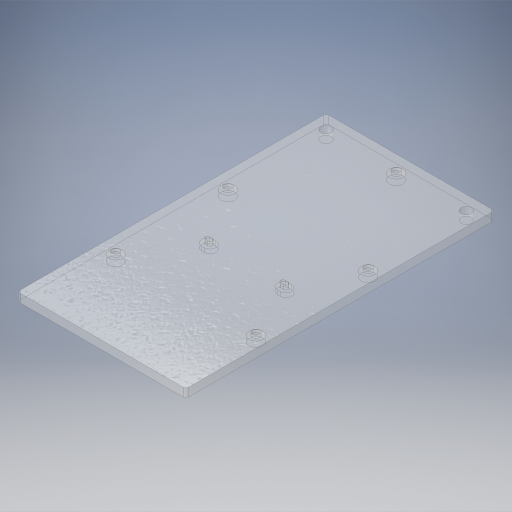
# Autodesk Inventor part: BT005_trajan20_21
Saved by Autodesk Inventor 2023 (Build 270158000, 158)
## iProperties
Company: HTBLA Kaindorf
RuleStatus: InUse
Created: 2022-08-07
Part Number: BT005_trajan20_21
Project: Zeichenmaschine_v2
Material: Acryl
Description: getriebemotor platte unten
Document SubType Name: Modeling
Designer: trajan20
Density: 1.188 g/cm^3
Appearance: Transparent - farblos
Mass: 184.772 g
Surface Area: 577.283 cm^2
Volume: 155.532 cm^3
AfterDocNew0: iProperties-Editor_aufrufen
Author: jan
Keywords: 2021
Autodesk Inventor part; units mm, degrees
ref_plane "YZ Plane" through (0, 0, 0) normal (1, 0, 0) x (0, 1, 0)
sketch "Skizze3" plane through (0, 0, 0) normal (0, 0, 1) x (1, 0, 0)
  line L0 (0, 0) -> (-220, 0)
  line L1 (-220, 0) -> (-220, 120)
  line L2 (-220, 120) -> (0, 120)
  line L3 (0, 120) -> (0, 0)
  point P0 (-210, 60)
  point P1 (-140, 10)
  point P2 (-140, 110)
  point P3 (-220, 60)
  point P4 (-60, 10)
  point P5 (-60, 110)
  point P6 (-210, 10)
  point P7 (-210, 110)
  dimension "d4" = 120
  dimension "d5" = 220
  dimension "d31" = 10
  dimension "d32" = 10
  dimension "d33" = 10
  dimension "d34" = 80
  dimension "d42" = 60
  constraints: 8 end point, 5 horizontal alignment, 4 vertical alignment, 2 parallel, 1 horizontal, 1 midpoint, 1 perpendicular
  measures "d4" distance between parallel lines of L0 L2
  measures "d5" distance between parallel lines of L1 L3
  measures "d31" distance from line of L1 point (-210, 60)
  measures "d32" distance from line of point (-140, 110) L2
  measures "d33" distance from line of L0 point (-140, 10)
  measures "d34" distance from line of L1 point (-140, 10)
  measures "d42" distance from line of L3 point (-60, 110)
extrude "Extrusion3" add sketch "Skizze3" along normal blind 6
ref_plane "Arbeitsebene1" through (-110, 120, 6) normal (-1, 0, 0) x (0, -1, 0)
ref_plane "Arbeitsebene2" through (-220, 60, 6) normal (0, -1, 0) x (1, 0, 0)
fillet "Rundung2" radius 2 4 edges at (0, 0, 3) (0, 120, 3) (-220, 120, 3) (-220, 0, 3)
derived "BT000_trajan20_22_Zeichenmaschine_neu_Masterskizze.ipt"
hole "Bohrung2" at (-210, 60, 0) at (-140, 10, 0) at (-140, 110, 0) at (-60, 110, 0) at (-60, 10, 0) direction (0, 0, 1) diameter 5.5 end through all counterbore diameter 10 counterbore depth 4
hole "Bohrung3" at (-210, 10, 0) at (-210, 110, 0) direction (0, 0, 1) diameter 7.5 end through all
derived "BT102_trajan20_21_Zeichenmaschine_v2_Platte Getriebemotor.ip"
sketch "Skizze6" plane through (0, 0, -6) normal (0, 0, -1) x (-1, 0, 0)
  circle A0 centre (60, 110) radius 2.75
  circle A1 centre (140, 10) radius 2.75
  circle A2 centre (60, 10) radius 2.75
  circle A3 centre (140, 110) radius 2.75
  circle A4 centre (210, 60) radius 2.75
  arc A5 (0, 2) -> (2, 0) centre (2, 2) ccw
  line L0 (2, 0) -> (218, 0)
  arc A6 (218, 0) -> (220, 2) centre (218, 2) ccw
  line L1 (220, 2) -> (220, 118)
  arc A7 (220, 118) -> (218, 120) centre (218, 118) ccw
  line L2 (218, 120) -> (2, 120)
  arc A8 (2, 120) -> (0, 118) centre (2, 118) ccw
  line L3 (0, 118) -> (0, 2)
  circle A9 centre (179.05, 69.25) radius 3.775
  line L4 (138.8, 76) -> (184.8, 76)
  line L5 (184.8, 76) -> (184.8, 44)
  circle A10 centre (179.05, 50.75) radius 3.775
  circle A11 centre (179.05, 50.75) radius 1.55
  line L6 (184.8, 44) -> (138.8, 44)
  line L7 (138.8, 44) -> (138.8, 76)
  circle A12 centre (145.55, 50.75) radius 3.775
  circle A13 centre (145.55, 50.75) radius 1.55
  circle A14 centre (145.55, 69.25) radius 3.775
  circle A15 centre (145.55, 69.25) radius 1.55
  circle A16 centre (170, 60) radius 6.675
  circle A17 centre (170, 60) radius 3.1
  circle A18 centre (179.05, 69.25) radius 1.55
  line L8 (123.8, 84) -> (192.8, 84)
  line L9 (192.8, 84) -> (192.8, 36)
  line L10 (192.8, 36) -> (123.8, 36)
  line L11 (123.8, 36) -> (123.8, 84)
  line L12 (138.8, 62.5) -> (103.8, 62.5)
  line L13 (138.8, 57.5) -> (103.8, 57.5)
  line L14 (103.8, 67.5) -> (138.8, 67.5)
  line L15 (138.8, 57.5) -> (103.8, 67.5)
  line L16 (103.8, 57.5) -> (138.8, 67.5)
  line L17 (97.7, 99.5) -> (103.8, 99.5)
  line L18 (97.7, 25.5) -> (97.7, 99.5)
  line L19 (97.7, 85.5) -> (47.7, 85.5)
  line L20 (47.7, 39.5) -> (97.7, 39.5)
  line L21 (103.8, 99.5) -> (103.8, 25.5)
  line L22 (103.8, 25.5) -> (97.7, 25.5)
  line L23 (47.7, 39.5) -> (47.7, 85.5)
  line L24 (119.8, 90.5) -> (119.8, 88.5)
  line L25 (118.2, 90.5) -> (118.2, 88.5)
  line L26 (121.4, 88.5) -> (121.4, 90.5)
  arc A19 (121.4, 90.5) -> (118.2, 90.5) centre (119.8, 90.5) ccw
  arc A20 (118.2, 88.5) -> (121.4, 88.5) centre (119.8, 88.5) ccw
  line L27 (119.8, 36.5) -> (119.8, 34.5)
  line L28 (118.2, 36.5) -> (118.2, 34.5)
  line L29 (121.4, 34.5) -> (121.4, 36.5)
  arc A21 (121.4, 36.5) -> (118.2, 36.5) centre (119.8, 36.5) ccw
  arc A22 (118.2, 34.5) -> (121.4, 34.5) centre (119.8, 34.5) ccw
  line L30 (103.8, 39.5) -> (108.8, 39.5)
  line L31 (108.8, 39.5) -> (108.8, 85.5)
  line L32 (108.8, 85.5) -> (95.8, 85.5)
  line L33 (159.9, 55) -> (159.9, 65)
  line L34 (153.7, 65) -> (153.7, 55)
  arc A23 (159.9, 65) -> (153.7, 65) centre (156.8, 65) ccw
  arc A24 (153.7, 55) -> (159.9, 55) centre (156.8, 55) ccw
  point P0 (0, 0)
  point P1 (138.8, 60)
  point P2 (123.8, 60)
  point P3 (121.3, 62.5)
  point P4 (92.3, 62.6)
  point P5 (95.8, 62.6)
  point P6 (97.7, 62.5)
  point P7 (47.7, 62.5)
  point P8 (119.8, 89.5)
  point P9 (119.8, 35.5)
  point P10 (100.75, 25.5)
  point P11 (102.3, 85.5)
sketch "Skizze5" plane through (0, 0, 0) normal (0, 0, -1) x (-1, 0, 0)
  line L0 (97.7, 25.5) -> (97.7, 99.5) projected
  line L1 (103.8, 99.5) -> (103.8, 25.5) projected
  line L2 (118.2, 36.5) -> (118.2, 34.5) projected
  arc A0 (121.4, 36.5) -> (118.2, 36.5) centre (119.8, 36.5) ccw projected
  line L3 (121.4, 34.5) -> (121.4, 36.5) projected
  arc A1 (118.2, 34.5) -> (121.4, 34.5) centre (119.8, 34.5) ccw projected
  line L4 (100.8, 88.4) -> (100.8, 90.6) construction
  line L5 (102.4, 88.4) -> (102.4, 90.6)
  line L6 (99.2, 90.6) -> (99.2, 88.4)
  arc A2 (99.2, 88.4) -> (102.4, 88.4) centre (100.8, 88.4) ccw
  arc A3 (102.4, 90.6) -> (99.2, 90.6) centre (100.8, 90.6) ccw
  circle A4 centre (210, 10) radius 3.75 projected
  circle A5 centre (210, 110) radius 3.75 projected
  circle A6 centre (60, 110) radius 5 projected
  circle A7 centre (140, 10) radius 5 projected
  circle A8 centre (210, 60) radius 5 projected
  circle A9 centre (140, 110) radius 5 projected
  circle A10 centre (60, 10) radius 5 projected
  arc A11 (218, 0) -> (220, 2) centre (218, 2) ccw projected
  line L7 (220, 118) -> (220, 2) projected
  arc A12 (220, 118) -> (218, 120) centre (218, 118) ccw projected
  line L8 (2, 120) -> (218, 120) projected
  arc A13 (2, 120) -> (0, 118) centre (2, 118) ccw projected
  line L9 (0, 2) -> (0, 118) projected
  arc A14 (0, 2) -> (2, 0) centre (2, 2) ccw projected
  line L10 (218, 0) -> (2, 0) projected
  line L11 (119.8, 36.5) -> (119.8, 34.5) projected
  line L12 (100.8, 34.5) -> (100.8, 36.5) construction
  line L13 (102.4, 34.5) -> (102.4, 36.5)
  line L14 (99.2, 36.5) -> (99.2, 34.5)
  arc A15 (99.2, 34.5) -> (102.4, 34.5) centre (100.8, 34.5) ccw
  arc A16 (102.4, 36.5) -> (99.2, 36.5) centre (100.8, 36.5) ccw
  arc A17 (121.4, 90.5) -> (118.2, 90.5) centre (119.8, 90.5) ccw projected
  line L15 (104.9, 88.4) -> (104.9, 90.6)
  arc A18 (104.9, 90.6) -> (96.7, 90.6) centre (100.8, 90.6) ccw
  line L16 (96.7, 90.6) -> (96.7, 88.4)
  arc A19 (96.7, 88.4) -> (104.9, 88.4) centre (100.8, 88.4) ccw
  line L17 (104.9, 36.5) -> (104.9, 34.5)
  arc A20 (96.7, 34.5) -> (104.9, 34.5) centre (100.8, 34.5) ccw
  line L18 (96.7, 34.5) -> (96.7, 36.5)
  arc A21 (104.9, 36.5) -> (96.7, 36.5) centre (100.8, 36.5) ccw
  point P0 (0, 0)
  point P1 (103.8, 90.6)
  point P2 (119.8, 35.5)
  point P3 (100.8, 89.5)
  point P4 (119.8, 89.5)
  point P5 (100.8, 35.5)
  point P6 (119.8, 35.5)
  dimension "d57" = 3.1
  dimension "d58" = 3.1
  dimension "d61" = 2.5
  dimension "d62" = 2.5
  constraints: 24 end point, 16 point on circle, 8 centre point, 8 tangent, 5 parallel, 4 horizontal alignment, 3 midpoint, 2 equal radius, 1 vertical, 6 other
  measures "d57" distance from line of L0 point (100.8, 89.5)
  measures "d58" distance from line of L0 point (100.8, 35.5)
  measures "d61" radial gap between concentric circles of A2 A19
  measures "d62" distance between parallel lines of L13 L17
extrude "Extrusion5" cut sketch "Skizze5" against normal through all contours A2 L6 A3 L5 | A15 L14 A16 L13
extrude "Extrusion6" cut sketch "Skizze5" against normal blind 3 contours A20 L18 A21 L0 | L0 A21 L1 A20 | L1 A21 L17 A20 | A19 L16 A18 L0 | L0 A18 L1 A19 | L1 A18 L15 A19
equation "\"d4\" = Basis_Zubau_Breite_Profillänge + 4 * AluProfil_Abstand"
equation "\"d5\" = Basis_Zubau_Länge_Profillänge + 2 * AluProfil_Abstand"
equation "\"d31\" = AluProfil_Abstand"
equation "\"d32\" = AluProfil_Abstand"
equation "\"d33\" = AluProfil_Abstand"
equation "\"d61\" = d62"
equation "\"Basis_Zubau_Breite_Profillänge\" = 80"
equation "\"AluProfil_Abstand\" = 10"
equation "\"Basis_Zubau_Länge_Profillänge\" = 200"
